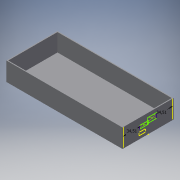
# Autodesk Inventor part: Bas
Saved by Autodesk Inventor 2019 (Build 230136000, 136)
## iProperties
Created: 2018-12-14
Part Number: Bas
Material: Generic
Document SubType Name: Modeling
Designer: Filip
Density: 1 g/cm^3
Appearance: Default
Author: Filip
Autodesk Inventor part; units mm, degrees
ref_plane "YZ Plane" through (0, 0, 0) normal (1, 0, 0) x (0, 1, 0)
ref_plane "XZ Plane" through (0, 0, 0) normal (0, 1, 0) x (-1, 0, 0)
ref_plane "XY Plane" through (0, 0, 0) normal (0, 0, 1) x (1, 0, 0)
sketch "Sketch1" plane through (0, 0, 0) normal (0, 1, 0) x (-1, 0, 0)
  line L0 (-125, -55) -> (125, -55)
  line L1 (125, -55) -> (125, 55)
  line L2 (125, 55) -> (-125, 55)
  line L3 (-125, 55) -> (-125, -55)
  line L4 (-125, -55) -> (125, 55) construction
  line L5 (125, -55) -> (-125, 55) construction
  point P0 (0, 0)
  dimension "d0" = 250
  dimension "d1" = 110
  constraints: 12 end point, 2 midpoint, 2 parallel, 1 horizontal, 1 perpendicular
  measures "d0" distance of L1.end L2.end
  measures "d1" distance of L0.end L1.end
extrude "Extrusion1" add sketch "Sketch1" along normal blind 40
shell "Shell1" thickness 2 removed faces 1 at (41.6667, 40, 18.3333)
sketch "Sketch2" plane through (125, 0, 55) normal (1, 0, 0) x (0, 0, -1)
  line L0 (2, 2) -> (2, 40) projected
  line L1 (108, 2) -> (108, 40) projected
  line L2 (36.5095, 25.828) -> (55.5893, 25.828)
  line L3 (55.5893, 25.828) -> (55.5893, 18.9836)
  line L4 (55.5893, 18.9836) -> (36.5095, 18.9836)
  line L5 (36.5095, 18.9836) -> (36.5095, 25.828)
  line L6 (36.5095, 25.828) -> (55.5893, 18.9836) construction
  line L7 (55.5893, 25.828) -> (36.5095, 18.9836) construction
  line L8 (52.9744, 31.7083) -> (73.4905, 31.7083)
  line L9 (73.4905, 31.7083) -> (73.4905, 21)
  line L10 (73.4905, 21) -> (52.9744, 21)
  line L11 (52.9744, 21) -> (52.9744, 31.7083)
  line L12 (52.9744, 31.7083) -> (73.4905, 21) construction
  line L13 (73.4905, 31.7083) -> (52.9744, 21) construction
  line L14 (48.1197, 13.67) -> (36.2802, 13.67) projected
  line L15 (34.9303, 8.35) -> (34.9303, 12.32) projected
  line L16 (49.4696, 12.32) -> (49.4696, 8.35) projected
  line L17 (36.0302, 7.3) -> (41.98, 7.3) projected
  line L18 (42.03, 7.3) -> (48.3697, 7.3) projected
  point P0 (55, 0)
  point P1 (46.0494, 22.4058)
  point P2 (63.2324, 26.3541)
  dimension "d5" = 34.5095
  dimension "d6" = 34.5095
  constraints: 24 end point, 4 midpoint, 4 parallel, 2 horizontal, 2 perpendicular
  measures "d5" distance between parallel lines of L5 L0
  measures "d6" distance between parallel lines of L9 L1
body "Solid1"
